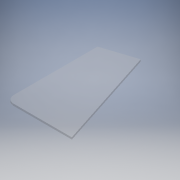
# Autodesk Inventor part: Gear Plates
Saved by Autodesk Inventor 2017 (Build 210142000, 142)
## iProperties
Created: 2017-01-12
Part Number: Gear Plates
Material: Generic
Document SubType Name: Modeling
Designer: Ben
Density: 1 g/cm^3
Appearance: Polycarbonate - Clear
Author: Ben
Autodesk Inventor part; units mm, degrees
ref_plane "YZ Plane" through (0, 0, 0) normal (1, 0, 0) x (0, 1, 0)
ref_plane "XZ Plane" through (0, 0, 0) normal (0, 1, 0) x (-1, 0, 0)
ref_plane "XY Plane" through (0, 0, 0) normal (0, 0, 1) x (1, 0, 0)
sketch "Sketch1" plane through (0, 0, 0) normal (0, 1, 0) x (-1, 0, 0)
  line L0 (0, 0) -> (0, 152.4)
  line L1 (0, 0) -> (-54.3529, -17.6603)
  line L2 (-54.3529, -17.6603) -> (-109.6088, 152.4)
  line L3 (0, 152.4) -> (-109.6088, 152.4)
  dimension "d0" = 72
  dimension "d1" = 152.4
  dimension "d2" = 57.15
  constraints: 8 end point, 2 perpendicular, 1 vertical
  measures "d0" angle of L0 L1
  measures "d1" distance of L0.start L0.end
  measures "d2" distance of L0.start L1.end
extrude "Extrusion1" add sketch "Sketch1" along normal blind 3.175
fillet "Fillet1" radius 12.7 1 edges at (0, 1.5875, 152.4)
body "Solid1"
